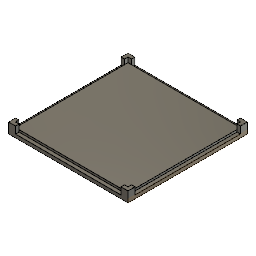
Plate-bottom (Autodesk Fusion 360 design; units mm, degrees)
Autodesk Fusion 360 part; units mm, degrees
note: some values were not read from the file. Chosen so that the rebuilt part matches the saved one: which pieces of a blend or face edit are solid.
sketch "Sketch1" plane through (0, 0, 0) normal (0, 1, 0) x (1, 0, 0)
  line L0 (-30, -40) -> (140, -40)
  line L1 (140, -40) -> (140, 130)
  line L2 (140, 130) -> (-30, 130)
  line L3 (-30, 130) -> (-30, -40)
  dimension "d1" = 170
  dimension "d2" = 170
  constraint horizontal L0
  constraint vertical L1
  constraint horizontal L2
  constraint vertical L3
  measures "d1" distance of L0.start L0.end
  measures "d2" distance of L0.start L2.end
extrude "Extrude1" add sketch "Sketch1" along normal blind 5
sketch "Sketch2" plane through (0, 5, 0) normal (0, 1, 0) x (-1, 0, 0)
  line L0 (30, -130) -> (30, 40)
  line L1 (30, 40) -> (-140, 40)
  line L2 (-140, 40) -> (-140, -130)
  line L3 (-140, -130) -> (30, -130)
  line L4 (30, -130) -> (20, -130)
  line L5 (20, -130) -> (20, -120)
  line L6 (20, -120) -> (30, -120)
  line L7 (30, -120) -> (30, -130)
  dimension "d5" = 10
  constraint horizontal L4
  constraint vertical L5
  constraint horizontal L6
  constraint vertical L7
  constraint coincident L0.start L3.end
  measures "d5" distance of L0.start L6.end
extrude "Extrude2" add sketch "Sketch2" along normal blind 10 contours L0 L3 L4 L5 L6 L7
sketch "Sketch3" plane through (0, 15, 0) normal (0, 1, 0) x (-1, 0, 0)
  line L0 (30, -120) -> (20, -120)
  line L1 (20, -120) -> (20, -130)
  line L2 (20, -130) -> (30, -130)
  line L3 (30, -130) -> (30, -120)
  line L4 (30, 40) -> (20, 40)
  line L5 (20, 40) -> (20, 30)
  line L6 (20, 30) -> (30, 30)
  line L7 (30, 30) -> (30, 40)
  point P0 (30, 40)
  constraint horizontal L4
  constraint vertical L5
  constraint horizontal L6
  constraint vertical L7
  constraint coincident P0 L4.start
sketch "Sketch4" plane through (140, 0, 0) normal (1, 0, 0) x (0, 0, -1)
  line L0 (-40, 0) -> (130, 0)
  line L1 (130, 0) -> (130, 5)
  line L2 (130, 5) -> (-40, 5)
  line L3 (-40, 5) -> (-40, 0)
sketch "Sketch5" plane through (0, 5, 0) normal (0, 1, 0) x (-1, 0, 0)
  line L0 (20, -130) -> (20, -120)
  line L1 (20, -120) -> (30, -120)
  line L2 (30, -120) -> (30, 40)
  line L3 (30, 40) -> (-140, 40)
  line L4 (-140, 40) -> (-140, -130)
  line L5 (-140, -130) -> (20, -130)
  line L6 (-140, -130) -> (-130, -130)
  line L7 (-130, -130) -> (-130, -120)
  line L8 (-130, -120) -> (-140, -120)
  line L9 (-140, -120) -> (-140, -130)
  dimension "d10" = 10
  constraint horizontal L6
  constraint vertical L7
  constraint horizontal L8
  constraint vertical L9
  constraint coincident L4.end L5.start
  measures "d10" distance of L4.end L6.end
extrude "Extrude4" add sketch "Sketch5" along normal blind 10 contours L4 L5 L6 L7 L8 L9
sketch "Sketch6" plane through (0, 5, 0) normal (0, 1, 0) x (-1, 0, 0)
  line L0 (-130, -120) -> (-130, -130)
  line L1 (-130, -130) -> (20, -130)
  line L2 (20, -130) -> (20, -120)
  line L3 (20, -120) -> (30, -120)
  line L4 (30, -120) -> (30, 40)
  line L5 (30, 40) -> (-140, 40)
  line L6 (-140, 40) -> (-140, -120)
  line L7 (-140, -120) -> (-130, -120)
  line L8 (-140, 40) -> (-130, 40)
  line L9 (-130, 40) -> (-130, 30)
  line L10 (-130, 30) -> (-140, 30)
  line L11 (-140, 30) -> (-140, 40)
  dimension "d13" = 10
  constraint horizontal L8
  constraint vertical L9
  constraint horizontal L10
  constraint vertical L11
  constraint coincident L5.end L6.start
  measures "d13" distance of L5.end L8.end
extrude "Extrude5" add sketch "Sketch6" along normal blind 10 contours L5 L6 L8 L9 L10 L11
sketch "Sketch7" plane through (0, 5, 0) normal (0, 1, 0) x (-1, 0, 0)
  line L0 (-130, 40) -> (-130, 30)
  line L1 (-130, 30) -> (-140, 30)
  line L2 (-140, 30) -> (-140, -120)
  line L3 (-140, -120) -> (-130, -120)
  line L4 (-130, -120) -> (-130, -130)
  line L5 (-130, -130) -> (20, -130)
  line L6 (20, -130) -> (20, -120)
  line L7 (20, -120) -> (30, -120)
  line L8 (30, -120) -> (30, 40)
  line L9 (30, 40) -> (-130, 40)
  line L10 (30, 40) -> (20, 40)
  line L11 (20, 40) -> (20, 30)
  line L12 (20, 30) -> (30, 30)
  line L13 (30, 30) -> (30, 40)
  constraint horizontal L10
  constraint vertical L11
  constraint horizontal L12
  constraint vertical L13
  constraint coincident L8.end L9.start
extrude "Extrude6" add sketch "Sketch7" along normal blind 10 contours L8 L9 L10 L11 L12 L13
sketch "Sketch8" plane through (0, 15, 0) normal (0, 1, 0) x (-1, 0, 0)
  line L0 (30, 30) -> (30, 40)
  line L1 (30, 40) -> (20, 40)
  line L2 (20, 40) -> (20, 30)
  line L3 (20, 30) -> (30, 30)
  line L4 (20, 30) -> (25, 30)
  line L5 (25, 30) -> (25, 35)
  line L6 (25, 35) -> (20, 35)
  line L7 (20, 35) -> (20, 30)
  constraint horizontal L4
  constraint vertical L5
  constraint horizontal L6
  constraint vertical L7
  constraint coincident L2.end L3.start
extrude "Extrude7" cut sketch "Sketch8" against normal blind 10 contours L2 L3 L4 L5 L6 L7
sketch "Sketch9" plane through (0, 5, 0) normal (0, 1, 0) x (-1, 0, 0)
  line L0 (20, 35) -> (20, 40)
  line L1 (20, 40) -> (-130, 40)
  line L2 (-130, 40) -> (-130, 30)
  line L3 (-130, 30) -> (-140, 30)
  line L4 (-140, 30) -> (-140, -120)
  line L5 (-140, -120) -> (-130, -120)
  line L6 (-130, -120) -> (-130, -130)
  line L7 (-130, -130) -> (20, -130)
  line L8 (20, -130) -> (20, -120)
  line L9 (20, -120) -> (30, -120)
  line L10 (30, -120) -> (30, 30)
  line L11 (30, 30) -> (25, 30)
  line L12 (25, 30) -> (25, 35)
  line L13 (25, 35) -> (20, 35)
  line L14 (25, -125) -> (-135, -125)
  line L15 (-135, -125) -> (-135, 35)
  line L16 (-135, 35) -> (25, 35)
  line L17 (25, 35) -> (25, -125)
  constraint horizontal L14
  constraint vertical L15
  constraint horizontal L16
  constraint vertical L17
extrude "Extrude11" add sketch "Sketch9" along normal blind 3 contours L2 L3 L5 L6 L8 L9 L12 L13 L14 L15 L16 L17
sketch "Sketch10" plane through (0, 15, 0) normal (0, 1, 0) x (-1, 0, 0)
  line L0 (30, -120) -> (20, -120)
  line L1 (20, -120) -> (20, -130)
  line L2 (20, -130) -> (30, -130)
  line L3 (30, -130) -> (30, -120)
  line L4 (20, -120) -> (25, -120)
  line L5 (25, -120) -> (25, -125)
  line L6 (25, -125) -> (20, -125)
  line L7 (20, -125) -> (20, -120)
  dimension "d20" = 5
  constraint horizontal L4
  constraint vertical L5
  constraint horizontal L6
  constraint vertical L7
  constraint coincident L0.end L1.start
  measures "d20" distance of L0.end L6.end
extrude "Extrude8" cut sketch "Sketch10" against normal blind 10 contours L0 L1 L4 L5 L6 L7
sketch "Sketch11" plane through (0, 15, 0) normal (0, 1, 0) x (-1, 0, 0)
  line L0 (-140, -120) -> (-140, -130)
  line L1 (-140, -130) -> (-130, -130)
  line L2 (-130, -130) -> (-130, -120)
  line L3 (-130, -120) -> (-140, -120)
  line L4 (-135, -125) -> (-130, -125)
  line L5 (-130, -125) -> (-130, -120)
  line L6 (-130, -120) -> (-135, -120)
  line L7 (-135, -120) -> (-135, -125)
  constraint horizontal L4
  constraint vertical L5
  constraint horizontal L6
  constraint vertical L7
  constraint coincident L2.end L3.start
extrude "Extrude9" cut sketch "Sketch11" against normal blind 10 contours L2 L3 L4 L5 L6 L7
sketch "Sketch12" plane through (0, 15, 0) normal (0, 1, 0) x (-1, 0, 0)
  line L0 (-140, 30) -> (-130, 30)
  line L1 (-130, 30) -> (-130, 40)
  line L2 (-130, 40) -> (-140, 40)
  line L3 (-140, 40) -> (-140, 30)
  line L4 (-135, 35) -> (-130, 35)
  line L5 (-130, 35) -> (-130, 30)
  line L6 (-130, 30) -> (-135, 30)
  line L7 (-135, 30) -> (-135, 35)
  constraint horizontal L4
  constraint vertical L5
  constraint horizontal L6
  constraint vertical L7
  constraint coincident L0.end L1.start
extrude "Extrude10" cut sketch "Sketch12" against normal blind 10 contours L0 L1 L4 L5 L6 L7
extrude "Extrude12" add 1 faces at (133.3333, 5, 33.3333) along direction (0, 1, 0) blind 3
extrude "Extrude13" add 1 faces at (133.3333, 5, -121.6667) along direction (0, 1, 0) blind 3
extrude "Extrude14" add 1 faces at (-21.6667, 5, -121.6667) along direction (0, 1, 0) blind 3
sketch "Sketch14" plane through (0, 8, 0) normal (0, 1, 0) x (-1, 0, 0)
  line L0 (-135, 30) -> (-135, -120)
  line L1 (-135, -120) -> (-135, -125)
  line L2 (-135, -125) -> (-130, -125)
  line L3 (-130, -125) -> (20, -125)
  line L4 (20, -125) -> (25, -125)
  line L5 (25, -125) -> (25, -120)
  line L6 (25, -120) -> (25, 30)
  line L7 (25, 30) -> (25, 35)
  line L8 (25, 35) -> (20, 35)
  line L9 (20, 35) -> (-130, 35)
  line L10 (-130, 35) -> (-135, 35)
  line L11 (-135, 35) -> (-135, 30)
  circle A0 centre (-9.9955, 18.75) radius 1.25
  dimension "d37" = 2.5
  measures "d37" diameter of A0
extrude "Extrude15" add sketch "Sketch14" along normal blind 5 contours A0
delete_face "DeleteFace1" 1 faces at (8.747, 11.3333, 18.6877)
sketch "Sketch15" plane through (0, 13, 0) normal (0, 1, 0) x (-1, 0, 0)
sketch "Sketch13" plane through (0, 8, 0) normal (0, 1, 0) x (-1, 0, 0)
  line L0 (-135, 30) -> (-135, -120)
  line L1 (-135, -120) -> (-135, -125)
  line L2 (-135, -125) -> (-130, -125)
  line L3 (-130, -125) -> (20, -125)
  line L4 (20, -125) -> (25, -125)
  line L5 (25, -125) -> (25, -120)
  line L6 (25, -120) -> (25, 30)
  line L7 (25, 30) -> (25, 35)
  line L8 (25, 35) -> (20, 35)
  line L9 (20, 35) -> (-130, 35)
  line L10 (-130, 35) -> (-135, 35)
  line L11 (-135, 35) -> (-135, 30)
  line L12 (-10, -50) -> (-84.118, -50)
  line L13 (-84.118, -50) -> (-84.118, 18.58)
  line L14 (-84.118, 18.58) -> (-10, 18.58)
  line L15 (-10, 18.58) -> (-10, -50)
  circle A0 centre (-9.9955, 18.75) radius 1.25
  dimension "d35" = 74.118
  dimension "d36" = 68.58
  constraint horizontal L12
  constraint vertical L13
  constraint horizontal L14
  constraint vertical L15
  measures "d35" distance of L12.start L12.end
  measures "d36" distance of L12.start L14.end
